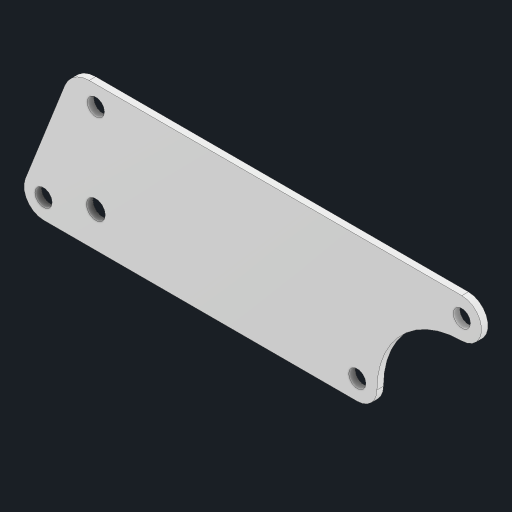
# Autodesk Inventor part: intake_base_outer
Saved by Autodesk Inventor 2024 (Build 280153000, 153)
## iProperties
Created: 2023-08-21
Part Number: intake_base_outer
Material: Acetal Resin, White
Document SubType Name: Modeling
Designer: Averey
Density: 1.425 g/cm^3
Appearance: Smooth - White
Author: Averey
Autodesk Inventor part; units mm, degrees
ref_plane "YZ Plane" through (0, 0, 0) normal (1, 0, 0) x (0, 1, 0)
ref_plane "XZ Plane" through (0, 0, 0) normal (0, 1, 0) x (-1, 0, 0)
ref_plane "XY Plane" through (0, 0, 0) normal (0, 0, 1) x (1, 0, 0)
sketch "Sketch1" plane through (0, 0, 0) normal (0, 0, 1) x (1, 0, 0)
  arc A0 (79.7785, -14.0465) -> (84.541, -9.284) centre (79.7785, -9.284) ccw
  circle A1 centre (3.5785, -9.284) radius 2.0955
  circle A2 centre (79.7785, -9.284) radius 2.0955
  arc A3 (84.541, 16.116) -> (79.7785, 20.8785) centre (79.7785, 16.116) ccw
  line L0 (23.4149, 20.8785) -> (79.7785, 20.8785)
  line L1 (84.541, 16.116) -> (84.541, -9.284)
  line L2 (79.7785, -14.0465) -> (3.5785, -14.0465)
  arc A4 (3.4793, -14.0455) -> (3.5785, -14.0465) centre (3.5785, -9.284) ccw
  arc A5 (-0.8541, -7.5424) -> (3.5785, -14.0465) centre (3.5785, -9.284) ccw
  line L3 (-0.8541, -7.5424) -> (8.7305, 16.8507)
  line L4 (23.4149, 20.8785) -> (14.6406, 20.8785)
  arc A6 (14.6406, 20.8785) -> (8.7305, 16.8507) centre (14.6406, 14.5285) ccw
  circle A7 centre (79.7785, 16.116) radius 2.0955
  point P0 (0, 0)
  point P1 (3.4793, -14.0455)
  dimension "d1" = 4.191
  dimension "d5" = 9.525
  dimension "d6" = 6.35
  dimension "d9" = 4.191
  constraints: 10 end point, 10 point on circle, 8 centre point, 6 tangent, 4 coincident, 1 horizontal, 1 perpendicular, 2 other
  measures "d1" diameter of A2
  measures "d5" diameter of A4
  measures "d6" radius of A6
  measures "d9" diameter of A7
extrude "Extrusion1" add sketch "Sketch1" along normal blind 1.5875 contours L2 A4 A5 L3 A6 L4 L0 A3 L1 A0 | A7
sketch "Sketch2" plane through (41.6785, -9.284, 1.5875) normal (0, 0, 1) x (1, 0, 0)
  arc A0 (42.8625, 25.4) -> (38.1, 30.1625) centre (38.1, 25.4) ccw projected
  circle A1 centre (63.5, 25.4) radius 2.0955
  arc A2 (66.8676, 22.0324) -> (63.5, 30.1625) centre (63.5, 25.4) ccw
  line L0 (38.1, 30.1625) -> (63.5, 30.1625)
  arc A3 (38.1, -4.7625) -> (42.8625, 0) centre (38.1, 0) ccw projected
  line L1 (38.1, 30.1625) -> (-27.0379, 30.1625) projected
  line L2 (38.1, 30.1625) -> (35.3924, 30.1625)
  arc A4 (38.1, -4.7625) -> (41.4676, -3.3676) centre (38.1, 0) ccw
  line L3 (41.4676, -3.3676) -> (38.1, 30.1625)
  circle A5 centre (-25.4, 25.4) radius 2.0955
  circle A6 centre (38.1, 0) radius 2.0955 projected
  arc A7 (41.4676, -3.3676) -> (42.8625, 0) centre (38.1, 0) ccw
  arc A8 (63.5, 20.6375) -> (63.5, 30.1625) centre (63.5, 25.4) ccw
  arc A9 (63.5, 20.6375) -> (42.8625, 0) centre (63.5, 0) ccw
  circle A10 centre (-25.4, 3.81) radius 2.3114
  point P0 (-41.6785, 9.284)
  point P1 (66.8676, 22.0324)
  dimension "d15" = 9.525
  dimension "d18" = 4.191
  dimension "d22" = 4.6228
  constraints: 13 point on circle, 8 centre point, 6 end point, 3 coincident, 3 tangent, 2 concentric, 1 point on line, 1 other
  measures "d15" diameter of A2
  measures "d18" diameter of A5
  measures "d22" diameter of A10
extrude "Extrusion3" add sketch "Sketch2" against normal blind 1.5875 contours A8 A9 A3 L3 L0 A2
extrude "Extrusion4" cut sketch "Sketch2" against normal blind 1.5875 contours A5 | A10
body "Solid1"
